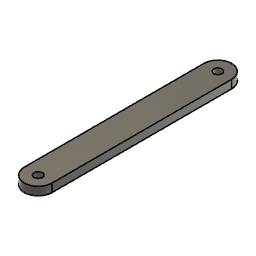
Double Door Opener 1 v2 (Autodesk Fusion 360 design; units mm, degrees)
Autodesk Fusion 360 part; units mm, degrees
sketch "Sketch1" plane through (0, 0, 0) normal (0, 1, 0) x (1, 0, 0)
  line L0 (5, 32.5) -> (-5, 32.5)
  line L1 (-5, 32.5) -> (-5, -32.5)
  line L2 (-5, -32.5) -> (5, -32.5)
  line L3 (5, -32.5) -> (5, 32.5)
  line L4 (5, 32.5) -> (-5, -32.5) construction
  line L5 (-5, 32.5) -> (5, -32.5) construction
  arc A0 (5, 32.5) -> (-5, 32.5) centre (0, 32.5) ccw
  line L6 (-5, 0) -> (5, 0) construction
  circle A1 centre (0, 32.5) radius 1.5
  arc A2 (-5, -32.5) -> (5, -32.5) centre (0, -32.5) ccw
  circle A3 centre (0, -32.5) radius 1.5
  dimension "d1" = 10
  dimension "d2" = 65
  dimension "d3" = 3
  constraint horizontal L0
  constraint perpendicular L0 L1
  constraint parallel L0 L2
  constraint parallel L1 L3
  constraint coincident L4 origin
  constraint coincident L5 origin
  constraint tangent L3 A0
  constraint midpoint L1 L6.start
  constraint midpoint L3 L6.end
  constraint concentric A0 A1
  constraint symmetric L0.start L6 L2.end
  constraint symmetric L0.end L6 L1.end
  constraint symmetric A0 L6 A2
  constraint symmetric L6 A1 A3
  measures "d1" distance of L1 L3
  measures "d2" distance of L0.end L1.end
  measures "d3" diameter of A1
extrude "Extrude1" add sketch "Sketch1" along normal blind 3 contours L0 L1 L2 L3 A1 A3 | L0 A0 A1 | L2 A2 A3
